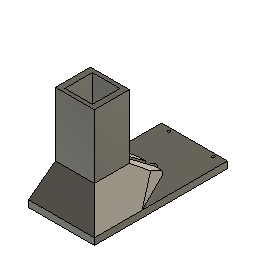
Camera_beacon (Autodesk Fusion 360 archive; units mm, degrees)
design "Postolje_beacon"
part number: 2026-02-18-15-47-36-932
Autodesk Fusion 360 part; units mm, degrees
sketch "Sketch1" plane through (0, 0, 0) normal (0, 0, 1) x (1, 0, 0)
  line L0 (21, -21) -> (-21, -21)
  line L1 (-21, -21) -> (-21, 21)
  line L2 (-21, 21) -> (21, 21)
  line L3 (21, 21) -> (21, -21)
  line L4 (21, -21) -> (-21, 21) construction
  line L5 (-21, -21) -> (21, 21) construction
  line L6 (29, 26) -> (-29, 26)
  line L7 (-29, 26) -> (-29, -26)
  line L8 (-29, -26) -> (29, -26)
  line L9 (29, -26) -> (29, 26)
  line L10 (29, 26) -> (-29, -26) construction
  line L11 (-29, 26) -> (29, -26) construction
  line L12 (0, 0) -> (37, 0)
  line L13 (0, 0) -> (-37, 0)
  line L14 (0, 0) -> (0, 37)
  circle A0 centre (37, 0) radius 2.5
  circle A1 centre (0, 37) radius 2.5
  circle A2 centre (-37, 0) radius 2.5
  line L15 (29, 0) -> (29, -10)
  line L16 (29, -10) -> (53, -10)
  line L17 (53, -10) -> (53, 10)
  line L18 (53, 10) -> (29, 10)
  line L19 (29, 10) -> (29, -10)
  line L20 (0, 26) -> (-10, 26)
  line L21 (-10, 26) -> (10, 26)
  line L22 (10, 26) -> (10, 50)
  line L23 (10, 50) -> (-10, 50)
  line L24 (-10, 50) -> (-10, 26)
  line L25 (-29, 0) -> (-29, -10)
  line L26 (-29, -10) -> (-53, -10)
  line L27 (-53, -10) -> (-53, 10)
  line L28 (-53, 10) -> (-29, 10)
  line L29 (-29, 10) -> (-29, -10)
  dimension "d28" = 24
  dimension "d29" = 24
  dimension "d30" = 24
  constraint horizontal L0
  constraint perpendicular L0 L1
  constraint parallel L0 L2
  constraint parallel L1 L3
  constraint coincident L4 L12.start
  constraint coincident L5 L12.start
  constraint coincident L12.start L13.start
  constraint horizontal L6
  constraint perpendicular L6 L7
  constraint parallel L6 L8
  constraint parallel L7 L9
  constraint coincident L10 L12.start
  constraint coincident L11 L12.start
  constraint perpendicular L3 L12
  constraint horizontal L13
  constraint perpendicular L2 L14
  constraint coincident L12.end A0.centre
  constraint coincident L14.end A1.centre
  constraint coincident L13.end A2.centre
  constraint midpoint L9 L15.start
  constraint coincident L9 L15.end
  constraint horizontal L16
  constraint vertical L17
  constraint horizontal L18
  constraint vertical L19
  constraint midpoint L6 L20.start
  constraint coincident L6 L20.end
  constraint horizontal L21
  constraint vertical L22
  constraint horizontal L23
  constraint vertical L24
  constraint midpoint L7 L25.start
  constraint coincident L7 L25.end
  constraint horizontal L26
  constraint vertical L27
  constraint horizontal L28
  constraint vertical L29
  measures "d28" distance of L25.end L26.end
  measures "d29" distance of L20.end L23.end
  measures "d30" distance of L17.end L18.end
extrude "Extrude1" add sketch "Sketch1" along normal blind 150 contours L0 L1 L3 L7 L8 L9 L12 L13 L15 L19 L25 L29 | L2 L3 L6 L9 L12 L14 L19 L21 | L1 L2 L6 L7 L13 L14 L20 L21 L29
extrude "Extrude2" add sketch "Sketch1" along normal blind 5 contours L9 L15 L16 L17 L18 L19 | L7 L25 L26 L27 L28 L29 | L6 L20 L21 L22 L23 L24
extrude "Extrude3" add 1 faces at (3.3333, 50, 1.6667) along direction (0, 1, 0) blind 102
extrude "Extrude4" add 1 faces at (10, 110, 3.3333) along direction (1, 0, 0) blind 43
extrude "Extrude5" add 1 faces at (-10, 110, 1.6667) along direction (-1, 0, 0) blind 43
extrude "Extrude6" add 2 faces at (37, -10, 1.6667) (-37, -10, 1.6667) along direction (0, -1, 0) blind 16
extrude "Extrude7" add 2 faces at (-45, 10, 3.3333) (45, 10, 1.6667) along direction (0, 1, 0) blind 16
extrude "Extrude9" add sketch "Sketch1" along normal blind 5 contours A0 | A1 | A2
sketch "Sketch2" plane through (0, 0, 5) normal (0, 0, 1) x (-1, 0, 0)
  line L0 (-29, 26) -> (-53, 26)
  line L1 (-53, 26) -> (-53, -152)
  line L2 (-53, -152) -> (53, -152)
  line L3 (53, -152) -> (53, 26)
  circle A0 centre (0, -60) radius 5
  circle A1 centre (0, -90) radius 5
  line L4 (-5, -60) -> (-5, -90)
  line L5 (5, -60) -> (5, -90)
  line L6 (-53, -152) -> (53, -152)
  line L7 (53, -152) -> (53, -142)
  line L8 (53, -142) -> (-53, -142)
  line L9 (-53, -142) -> (-53, -152)
  line L10 (29, -26) -> (-29, -26)
  line L11 (-29, -26) -> (-29, 26)
  line L12 (53, 26) -> (29, 26)
  line L13 (29, 26) -> (29, -26)
  circle A2 centre (-33, -147) radius 2
  circle A3 centre (33, -147) radius 2
  line L14 (35, -60) -> (35, -90)
  line L15 (25, -60) -> (25, -90)
  circle A4 centre (30, -60) radius 5
  circle A5 centre (30, -90) radius 5
  line L16 (-25, -60) -> (-25, -90)
  line L17 (-35, -60) -> (-35, -90)
  circle A6 centre (-30, -60) radius 5
  circle A7 centre (-30, -90) radius 5
  dimension "d45" = 10
  dimension "d46" = 10
  dimension "d64" = 4
  dimension "d65" = 4
  dimension "d70" = 10
  dimension "d71" = 10
  dimension "d72" = 10
  dimension "d73" = 10
  constraint coincident A0 L4.start
  constraint coincident A1 L4.end
  constraint tangent A1 L4
  constraint parallel L1 L4
  constraint coincident A0 L5.start
  constraint coincident A1 L5.end
  constraint tangent A1 L5
  constraint parallel L4 L5
  constraint horizontal L6
  constraint vertical L7
  constraint horizontal L8
  constraint vertical L9
  constraint coincident L1.end L2.start
  constraint coincident L15.start A4
  constraint coincident L15.end A5
  constraint tangent L15 A5
  constraint coincident L14.start A4
  constraint coincident L14.end A5
  constraint tangent L14 A5
  constraint parallel L14 L15
  constraint coincident L17.start A6
  constraint coincident L17.end A7
  constraint tangent L17 A7
  constraint coincident L16.start A6
  constraint coincident L16.end A7
  constraint tangent L16 A7
  constraint parallel L16 L17
  measures "d45" diameter of A0
  measures "d46" diameter of A1
  measures "d64" diameter of A2
  measures "d65" diameter of A3
  measures "d70" diameter of A4
  measures "d71" diameter of A5
  measures "d72" diameter of A6
  measures "d73" diameter of A7
extrude "Extrude10" cut sketch "Sketch2" against normal blind 10 contours A0 | A0 A1 L4 L5 | A1
sketch "Sketch3" plane through (0, -26, 0) normal (0, -1, 0) x (1, 0, 0)
  line L0 (-53, 0) -> (53, 0)
  line L1 (53, 0) -> (53, 5)
  line L2 (53, 5) -> (29, 5)
  line L3 (29, 5) -> (29, 150)
  line L4 (29, 150) -> (-29, 150)
  line L5 (-29, 150) -> (-29, 5)
  line L6 (-53, 5) -> (-53, 0)
  line L7 (-53, 5) -> (53, 5)
  line L8 (53, 5) -> (53, 0)
  line L9 (53, 0) -> (-53, 0)
  line L10 (-53, 0) -> (-53, 5)
  line L11 (-29, 5) -> (-53, 5)
  constraint horizontal L7
  constraint vertical L8
  constraint horizontal L9
  constraint vertical L10
  constraint coincident L0.end L1.start
  constraint coincident L6.start L7.start
extrude "Extrude12" add sketch "Sketch3" along normal blind 20 contours L0 L1 L2 L6 L7 L8 L9 L10 L11
chamfer "Chamfer1" distance 50 distance2 20 3 edges at (-29, 0, 5) (0, -26, 5) (29, 0, 5) measured on face at (-29, -8.6667, 101.6667) measured on face at (-9.6667, -26, 53.3333) measured on face at (29, -8.6667, 101.6667)
extrude "Extrude13" cut 1 faces at (-53, 110, 3.3333) along direction (1, 0, 0) blind 4
extrude "Extrude14" cut 1 faces at (53, 20, 3.3333) along direction (-1, 0, 0) blind 4
extrude "Extrude15" cut sketch "Sketch2" against normal blind 5 contours A2 | A3
extrude "Extrude16" add 1 faces at (-34.3333, 89.3333, 0) along direction (0, 0, -1) blind 5
sketch "Sketch4" plane through (0, 26, 0) normal (0, 1, 0) x (-1, 0, 0)
  line L0 (29, 55) -> (29, 150)
  line L1 (29, 150) -> (-29, 150)
  line L2 (-29, 150) -> (-29, 55)
  circle A0 centre (0, 100) radius 2.5
  circle A1 centre (0, 85) radius 2.5
  line L3 (-49, 5) -> (49, 5)
  line L4 (49, 5) -> (29, 55)
  line L5 (-29, 55) -> (-49, 5)
  dimension "d76" = 5
  dimension "d77" = 5
  measures "d76" diameter of A0
  measures "d77" diameter of A1
extrude "Extrude18" cut sketch "Sketch4" against normal blind 5 contours A0 | A1
extrude "Extrude19" add 1 faces at (7, -21, 98.3333) along direction (0, 1, 0) blind 0.5
extrude "Extrude20" add 1 faces at (0.0623, 21, 24.169) along direction (0, -1, 0) blind 0.5
extrude "Extrude21" add 1 faces at (21, 6.8333, 98.3333) along direction (-1, 0, 0) blind 0.5
extrude "Extrude22" add 1 faces at (-21, 6.8333, 98.3333) along direction (1, 0, 0) blind 0.5
sketch "Sketch5" plane through (0, 0, 5) normal (0, 0, 1) x (-1, 0, 0)
  circle A0 centre (-33, -147) radius 2
  circle A1 centre (33, -147) radius 2
  line L0 (-49, -26) -> (-49, -152)
  line L1 (-49, -152) -> (49, -152)
  line L2 (49, -152) -> (49, -26)
  line L3 (49, -26) -> (-49, -26)
  arc A2 (-5, -90) -> (5, -90) centre (0, -90) ccw
  line L4 (-5, -90) -> (-5, -60)
  arc A3 (5, -60) -> (-5, -60) centre (0, -60) ccw
  line L5 (5, -60) -> (5, -90)
  line L6 (-6.5, -90) -> (-18.5, -90)
  line L7 (-18.5, -90) -> (-18.5, -26)
  line L8 (-18.5, -26) -> (-6.5, -26)
  line L9 (-6.5, -26) -> (-6.5, -90)
  line L10 (6.5, -90) -> (18.5, -90)
  line L11 (18.5, -90) -> (18.5, -26)
  line L12 (18.5, -26) -> (6.5, -26)
  line L13 (6.5, -26) -> (6.5, -90)
  dimension "d92" = 12
  dimension "d93" = 12
  constraint horizontal L6
  constraint vertical L7
  constraint horizontal L8
  constraint vertical L9
  constraint horizontal L10
  constraint vertical L11
  constraint horizontal L12
  constraint vertical L13
  measures "d92" distance of L6.start L6.end
  measures "d93" distance of L10.start L10.end
extrude "Extrude23" add sketch "Sketch5" along normal blind 5 contours L3 L6 L7 L8 L9 | L3 L10 L11 L12 L13
chamfer "Chamfer3" distance 45 distance2 60 2 edges at (-12.5, 26, 10) (12.5, 26, 10) measured on face at (0.0623, 26, 134.1643) measured on face at (0.0623, 26, 134.1643)
extrude "Extrude24" cut 2 faces at (10.5, 90, 6.6667) (-10.5, 90, 6.6667) along direction (0, -1, 0) blind 4
chamfer "Chamfer5" distance 30 distance2 60 2 edges at (18.5, 26, 30) (-18.5, 26, 30) measured on face at (-0.0623, 26, 134.1643) measured on face at (-0.0623, 26, 134.1643)

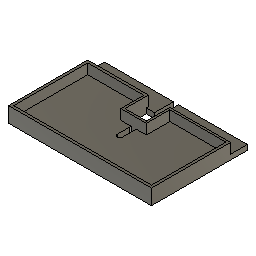
design "Beacon_kamera_postolje"
part number: 2026-02-18-16-44-35-691
Autodesk Fusion 360 part; units mm, degrees
sketch "Sketch1" plane through (0, 0, 0) normal (0, 0, 1) x (1, 0, 0)
  line L0 (21, -21) -> (-21, -21)
  line L1 (-21, -21) -> (-21, 21)
  line L2 (-21, 21) -> (21, 21)
  line L3 (21, 21) -> (21, -21)
  line L4 (21, -21) -> (-21, 21) construction
  line L5 (-21, -21) -> (21, 21) construction
  line L6 (0, 50) -> (0, -40)
  line L7 (-140, 50) -> (140, 50)
  line L8 (140, 50) -> (140, -130)
  line L9 (140, -130) -> (-140, -130)
  line L10 (-140, -130) -> (-140, 50)
  line L11 (-140, 50) -> (140, -130) construction
  line L12 (140, 50) -> (-140, -130) construction
  point P0 (0, -40)
  dimension "d1" = 42
  dimension "d2" = 42
  dimension "d14" = 280
  constraint horizontal L0
  constraint perpendicular L0 L1
  constraint parallel L0 L2
  constraint parallel L1 L3
  constraint coincident L4 origin
  constraint coincident L5 origin
  constraint perpendicular L0 L6
  constraint horizontal L7
  constraint perpendicular L7 L8
  constraint parallel L7 L9
  constraint parallel L8 L10
  constraint coincident L11 P0
  constraint coincident L12 P0
  constraint coincident P0 L6.end
  measures "d1" distance of L1.end L2.end
  measures "d2" distance of L0.end L1.end
  measures "d14" distance of L8.end L9.end
extrude "Extrude4" add sketch "Sketch1" along normal blind 10
sketch "Sketch3" plane through (0, 0, 10) normal (0, 0, 1) x (-1, 0, 0)
  line L0 (21, -21) -> (-21, -21)
  line L1 (-21, -21) -> (-21, 21)
  line L2 (-21, 21) -> (21, 21)
  line L3 (21, 21) -> (21, -21)
  line L4 (140, 130) -> (-140, 130)
  line L5 (-140, 130) -> (-140, -50)
  line L6 (-140, -50) -> (140, -50)
  line L7 (140, -50) -> (140, 130)
  line L8 (-120, 120) -> (40, 120)
  line L9 (40, 120) -> (40, 35)
  line L10 (40, 35) -> (-120, 35)
  line L11 (-120, 35) -> (-120, 120)
  line L12 (70, 100) -> (126, 100)
  line L13 (126, 100) -> (126, 15)
  line L14 (126, 15) -> (70, 15)
  line L15 (70, 15) -> (70, 100)
  line L16 (-140, -50) -> (-135, -50)
  line L17 (-135, -50) -> (-135, 130)
  line L18 (-135, 130) -> (-140, 130)
  line L19 (-140, 130) -> (-140, -50)
  line L20 (-135, 130) -> (140, 130)
  line L21 (140, 130) -> (140, 125)
  line L22 (140, 125) -> (-135, 125)
  line L23 (-135, 125) -> (-135, 130)
  line L24 (140, 125) -> (135, 125)
  line L25 (135, 125) -> (135, -25)
  line L26 (135, -25) -> (140, -25)
  line L27 (140, -25) -> (140, 125)
  line L28 (135, -25) -> (25, -25)
  line L29 (25, -25) -> (25, -20)
  line L30 (25, -20) -> (135, -20)
  line L31 (135, -20) -> (135, -25)
  line L32 (25, -25) -> (-25, -25)
  line L33 (-25, -25) -> (-25, 25)
  line L34 (-25, 25) -> (25, 25)
  line L35 (25, 25) -> (25, -25)
  line L36 (25, -25) -> (-25, 25) construction
  line L37 (-25, -25) -> (25, 25) construction
  line L38 (-25, -25) -> (-135, -25)
  line L39 (-25, -21) -> (-135, -21)
  dimension "d17" = 160
  dimension "d18" = 85
  dimension "d19" = 56
  dimension "d20" = 85
  dimension "d24" = 5
  dimension "d25" = 5
  dimension "d26" = 5
  dimension "d29" = 50
  dimension "d30" = 50
  constraint horizontal L8
  constraint vertical L9
  constraint horizontal L10
  constraint vertical L11
  constraint horizontal L12
  constraint vertical L13
  constraint horizontal L14
  constraint vertical L15
  constraint horizontal L16
  constraint vertical L17
  constraint horizontal L18
  constraint vertical L19
  constraint coincident L5.end L6.start
  constraint horizontal L20
  constraint vertical L21
  constraint horizontal L22
  constraint vertical L23
  constraint horizontal L24
  constraint vertical L25
  constraint horizontal L26
  constraint vertical L27
  constraint horizontal L28
  constraint vertical L29
  constraint horizontal L30
  constraint vertical L31
  constraint horizontal L32
  constraint perpendicular L32 L33
  constraint parallel L32 L34
  constraint parallel L33 L35
  constraint coincident L36 origin
  constraint coincident L37 origin
  constraint coincident L17 L38.end
  constraint perpendicular L17 L38
  constraint coincident L33 L39.start
  constraint coincident L17 L39.end
  constraint perpendicular L17 L39
  measures "d17" distance of L8.start L8.end
  measures "d18" distance of L8.start L10.end
  measures "d19" distance of L12.start L12.end
  measures "d20" distance of L12.start L14.end
  measures "d24" distance of L17.end L22.end
  measures "d25" distance of L21.end L24.end
  measures "d26" distance of L25.end L30.end
  measures "d29" distance of L33.end L34.end
  measures "d30" distance of L32.end L33.end
extrude "Extrude6" add sketch "Sketch3" along normal blind 10 contours L4 L7 L17 L20 L21 L22 L23 L24 | L4 L5 L6 L16 L17 L18 L19 L23 | L7 L22 L24 L25 L26 L27 L31 | L25 L28 L29 L30 L31 L35
extrude "Extrude7" add sketch "Sketch3" along normal blind 10 contours L29 L32 L33 L34 L35
extrude "Extrude8" add sketch "Sketch3" along normal blind 10 contours L17 L33 L38 L39
sketch "Sketch4" plane through (0, 50, 0) normal (0, 1, 0) x (-1, 0, 0)
  line L0 (-140, 0) -> (140, 0)
  line L1 (140, 0) -> (140, 10)
  line L2 (140, 10) -> (-135, 10)
  line L3 (-135, 10) -> (-135, 20)
  line L4 (-135, 20) -> (-140, 20)
  line L5 (-140, 20) -> (-140, 0)
  line L6 (-140, 10) -> (-135, 10)
  constraint midpoint L5 L6.start
  constraint coincident L2.end L3.start
extrude "Extrude9" cut sketch "Sketch4" against normal blind 25 contours L3 L4 L5 L6
extrude "Extrude10" add 1 faces at (45, -128.3333, 20) along direction (0, 0, 1) blind 10
sketch "Sketch6" plane through (0, 0, 10) normal (0, 0, 1) x (-1, 0, 0)
  line L0 (-135, -21) -> (-25, -21)
  line L1 (-25, -21) -> (-25, 25)
  line L2 (-25, 25) -> (25, 25)
  line L3 (25, 25) -> (25, -20)
  line L4 (25, -20) -> (135, -20)
  line L5 (135, -20) -> (135, 125)
  line L6 (135, 125) -> (-135, 125)
  line L7 (-135, 125) -> (-135, -21)
  line L8 (0, 21) -> (0, 28)
  line L9 (0, 28) -> (0, 52)
  circle A0 centre (0, 28) radius 5
  circle A1 centre (0, 28) radius 7
  circle A2 centre (0, 52) radius 5
  circle A3 centre (0, 52) radius 7
  line L10 (7, 28) -> (7, 52)
  line L11 (-7, 28) -> (-7, 51)
  line L12 (5, 28) -> (5, 52)
  line L13 (-5, 28) -> (-5, 52)
  line L14 (-5, -50) -> (5, -50)
  line L15 (5, -50) -> (5, -25)
  line L16 (5, -25) -> (-5, -25)
  line L17 (-5, -25) -> (-5, -50)
  dimension "d39" = 7
  dimension "d40" = 10
  dimension "d41" = 10
  dimension "d42" = 14
  constraint perpendicular L2 L8
  constraint parallel L8 L9
  constraint coincident L8.end L9.start
  constraint concentric A0 A1
  constraint coincident L8.start A1
  constraint coincident L9.end A2.centre
  constraint coincident A1 L10.start
  constraint coincident A3 L10.end
  constraint tangent A3 L10
  constraint coincident A1 L11.start
  constraint parallel L9 L11
  constraint coincident A0 L12.start
  constraint coincident A2 L12.end
  constraint tangent A2 L12
  constraint coincident A0 L13.start
  constraint coincident A2 L13.end
  constraint tangent A2 L13
  constraint horizontal L14
  constraint vertical L15
  constraint horizontal L16
  constraint vertical L17
  measures "d39" distance of L8.start L8.end
  measures "d40" diameter of A0
  measures "d41" diameter of A2
  measures "d42" diameter of A3
extrude "Extrude11" cut sketch "Sketch6" against normal blind 20 contours L2 L8 L9 A0 | L2 L8 L9 A0 | L9 A0 A1 L13 | L9 A1 A3 L13 | L9 A0 A1 L12 | L9 A1 A3 L12 | L9 A2 A3 L13 | L9 A2 A3 L12 | A2
extrude "Extrude12" cut sketch "Sketch6" against normal blind 20 contours L14 L15 L16 L17
sketch "Sketch7" plane through (0, 21, 0) normal (0, -1, 0) x (1, 0, 0)
  line L0 (-21, 0) -> (21, 0)
  line L1 (21, 0) -> (21, 30)
  line L2 (21, 30) -> (-21, 30)
  line L3 (-21, 30) -> (-21, 0)
  line L4 (-21, 30) -> (21, 30)
  line L5 (21, 30) -> (21, 10)
  line L6 (21, 10) -> (-21, 10)
  line L7 (-21, 10) -> (-21, 30)
  dimension "d47" = 20
  constraint horizontal L4
  constraint vertical L5
  constraint horizontal L6
  constraint vertical L7
  constraint coincident L2.end L3.start
  measures "d47" distance of L2.end L6.end
extrude "Extrude13" cut sketch "Sketch7" against normal blind 10 contours L1 L2 L3 L4 L5 L6 L7
extrude "Extrude14" cut 1 faces at (1.6667, 25, 3.3333) along direction (0, -1, 0) blind 5
extrude "Extrude15" add 2 faces at (50, 50, 3.3333) (-50, 50, 6.6667) along direction (0, 1, 0) blind 8
